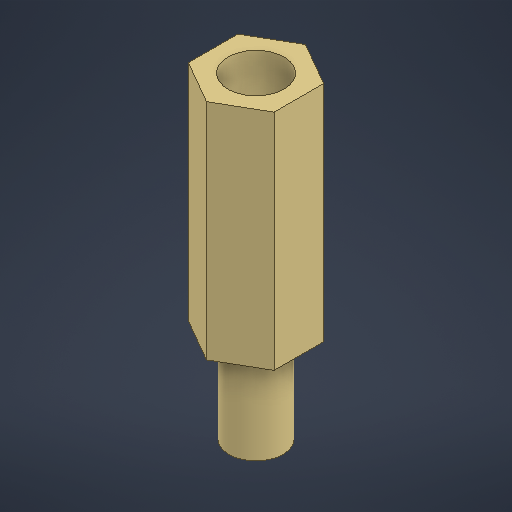
# Autodesk Inventor part: mounting
Saved by Autodesk Inventor 2025.2 (Build 292293000, 293)
## iProperties
Created: 2025-10-21
Part Number: mounting
Material: Generic
Document SubType Name: Modeling
Designer: micyg
Density: 1 g/cm^3
Appearance: Default
Author: micyg
Autodesk Inventor part; units mm, degrees
ref_plane "YZ Plane" through (0, 0, 0) normal (1, 0, 0) x (0, 1, 0)
ref_plane "XZ Plane" through (0, 0, 0) normal (0, 1, 0) x (-1, 0, 0)
ref_plane "XY Plane" through (0, 0, 0) normal (0, 0, 1) x (1, 0, 0)
sketch "Sketch1" plane through (0, 0, 0) normal (0, 1, 0) x (-1, 0, 0)
  line L0 (0, -2.6558) -> (-2.3, -1.3279)
  line L1 (-2.3, -1.3279) -> (-2.3, 1.3279)
  line L2 (-2.3, 1.3279) -> (0, 2.6558)
  line L3 (0, 2.6558) -> (2.3, 1.3279)
  line L4 (2.3, 1.3279) -> (2.3, -1.3279)
  line L5 (2.3, -1.3279) -> (0, -2.6558)
  circle A0 centre (0, 0) radius 1.45
  dimension "d4" = 2.9
  dimension "d5" = 4.6
  constraints: 12 end point, 2 coincident, 1 centre point, 13 other
  measures "d4" diameter of A0
  measures "d5" distance between parallel lines of L3 L0
extrude "Extrusion1" add sketch "Sketch1" along normal blind 12 contours L0 L1 L2 L3 L4 L5 | A0
extrude "Extrusion2" add sketch "Sketch1" against normal blind 5 contours A0
sketch "Sketch2" plane through (0, 12, 0) normal (0, 1, 0) x (1, 0, 0)
  circle A0 centre (0, 0) radius 1.45 projected
  circle A1 centre (0, 0) radius 1.45 projected
  circle A2 centre (0, 0) radius 1.5
  dimension "d6" = 3
  constraints: 1 centre point, 1 coincident
  measures "d6" diameter of A2
extrude "Extrusion3" cut sketch "Sketch2" against normal blind 10 contours A0 | A2
body "Solid1"
